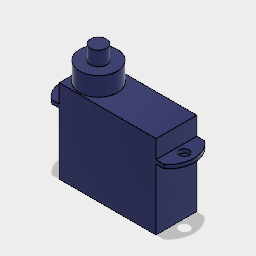
Pololu#1053 v4 (Autodesk Fusion 360 design; units mm, degrees)
Autodesk Fusion 360 part; units mm, degrees
note: some values were not read from the file. Set by a fixed rule: the direction of a hole.
sketch "Skizze1" plane through (0, 0, 0) normal (0, 1, 0) x (1, 0, 0)
  line L0 (0, 0) -> (20.2, 0)
  line L1 (20.2, 0) -> (20.2, -8.5)
  line L2 (20.2, -8.5) -> (0, -8.5)
  line L3 (0, -8.5) -> (0, 0)
  line L4 (0, 0) -> (-1.65, 0)
  line L5 (0, -8.5) -> (-1.65, -8.5)
  arc A0 (-1.65, 0) -> (-1.65, -8.5) centre (1.7305, -4.25) ccw
  line L6 (20.2, 0) -> (21.85, 0)
  line L7 (20.2, -8.5) -> (21.85, -8.5)
  arc A1 (21.85, -8.5) -> (21.85, 0) centre (18.4695, -4.25) ccw
  dimension "d1" = 20.2
  dimension "d2" = 8.5
  dimension "d3" = 1.65
  dimension "d4" = 3.95
  dimension "d5" = 1.65
  dimension "d6" = 1.65
  dimension "d7" = 3.7
  dimension "d8" = 1.65
  dimension "d9" = 1.65
  dimension "d10" = 1.65
  dimension "d11" = 3.7
  constraint horizontal L0
  constraint vertical L1
  constraint horizontal L2
  constraint vertical L3
  constraint coincident L0.start L3.end
  constraint perpendicular L3 L4
  constraint perpendicular L3 L5
  constraint coincident L0.start A0
  constraint perpendicular L1 L7
  constraint coincident L0.start A1
  measures "d5" distance of L0.start
extrude "Extrusion1" add sketch "Skizze1" along normal blind 0.8 contours L3 L4 L5 A0 makes body 1
extrude "Extrusion2" add sketch "Skizze1" along normal blind 0.8 separate body contours L1 L6 L7 A1 makes body 2
extrude "Extrusion3" add sketch "Skizze1" along normal blind 4.6 contours L0 L1 L2 L3 bodies 1 2
extrude "Extrusion4" add sketch "Skizze1" against normal blind 12.8 contours L0 L1 L2 L3 bodies 1
hole "Bohrung1" at (21.85, 0, 4.25) at (-1.65, 0, 4.25) direction (0, 1, 0) diameter 2 depth 1 tip angle 118 bodies 1
sketch "Skizze2" plane through (0, 4.6, 0) normal (0, 1, 0) x (-1, 0, 0)
  line L0 (0, 8.5) -> (-20.2, 8.5)
  line L1 (-20.2, 8.5) -> (-20.2, 0)
  line L2 (-20.2, 0) -> (0, 0)
  line L3 (0, 0) -> (0, 8.5)
  circle A0 centre (-3.95, 4.25) radius 3.95
  dimension "d23" = 7.9
  constraint coincident L2.end L3.start
  measures "d23" diameter of A0
extrude "Extrusion5" add sketch "Skizze2" along normal blind 3.9 contours A0 bodies 1
sketch "Skizze3" plane through (0, 8.5, 0) normal (0, 1, 0) x (-1, 0, 0)
  circle A0 centre (-3.95, 4.25) radius 3.95
  circle A1 centre (-3.95, 4.25) radius 1.7063
  constraint concentric A0 A1
extrude "Extrusion6" add sketch "Skizze3" along normal blind 3 contours A1 bodies 1
equation "d3 = ( ( 23.5 - 20.2 ) / 2 ) * 1 mm"
equation "d4 = 1.8 mm + ( ( 7.9 - 3.6 ) / 2 ) * 1 mm"
equation "d6 = d5"
equation "d8 = d5"
equation "d9 = d5"
equation "d10 = d3"
equation "d11 = d7"
